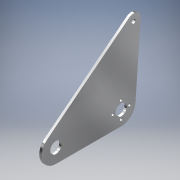
# Autodesk Inventor part: Module Plate
Saved by Autodesk Inventor 2019.4 (Build 234330000, 330)
## iProperties
Created: 2019-12-31
Part Number: Module Plate
Material: Aluminum 6061
Document SubType Name: Modeling
Designer: Mark
Mass: 136.058 g
Surface Area: 235.603 cm^2
Volume: 50.392 cm^3
Density: 2.7 g/cm^3
Appearance: Aluminum - Flat
Author: Mark
Autodesk Inventor part; units mm, degrees
ref_plane "YZ Plane" through (0, 0, 0) normal (1, 0, 0) x (0, 1, 0)
ref_plane "XZ Plane" through (0, 0, 0) normal (0, 1, 0) x (-1, 0, 0)
ref_plane "XY Plane" through (0, 0, 0) normal (0, 0, 1) x (1, 0, 0)
sketch "Sketch1" plane through (0, 0, 0) normal (1, 0, 0) x (0, 1, 0)
  circle A0 centre (0, 0) radius 12
  circle A1 centre (0, -137.4) radius 12
  line L0 (0, 0) -> (0, -137.4)
  line L1 (0, 0) -> (137.4, 0) construction
  line L2 (0, 0) -> (0, -137.4) construction
  line L3 (-30, 0) -> (-30, -137.4)
  line L4 (30, -137.4) -> (30, 0)
  arc A2 (30, 0) -> (-30, 0) centre (0, 0) ccw
  arc A3 (-30, -137.4) -> (30, -137.4) centre (0, -137.4) ccw
  circle A4 centre (0, -137.4) radius 17.5 construction
  line L5 (0, -137.4) -> (17.5, -137.4) construction
  line L6 (0, -137.4) -> (17.5, -137.4) construction
  circle A5 centre (17.5, -137.4) radius 2.65
  line L7 (0, -137.4) -> (0, -119.9) construction
  circle A6 centre (0, -119.9) radius 2.65
  line L8 (0, -137.4) -> (-17.5, -137.4) construction
  circle A7 centre (-17.5, -137.4) radius 2.65
  line L9 (0, -137.4) -> (0, -154.9) construction
  circle A8 centre (0, -154.9) radius 2.65
  line L10 (0, -137.4) -> (147.7212, -163.4472) construction
  line L11 (0, -137.4) -> (150, -137.4) construction
  circle A9 centre (147.7212, -163.4472) radius 5.1
  arc A10 (146.6067, -178.4058) -> (159.5086, -154.1705) centre (147.7212, -163.4472) ccw
  line L12 (146.6067, -178.4058) -> (-2.2289, -167.3171)
  line L13 (159.5086, -154.1705) -> (23.5748, 18.5534)
  point P0 (0, -68.7)
  point P1 (-20.8357, -21.5841)
  dimension "d9" = 35
  dimension "d0" = 24
  dimension "d1" = 24
  dimension "d4" = 90
  dimension "d5" = 137.4
  dimension "d6" = 60
  dimension "d10" = 0
  dimension "d11" = 5.3
  dimension "d14" = 360
  dimension "d16" = 150
  dimension "d17" = 350
  dimension "d18" = 10.2
  dimension "d19" = 30
  constraints: 30 end point, 10 centre point, 9 point on circle, 8 tangent, 5 coincident, 3 equal length, 3 horizontal, 2 vertical, 1 horizontal alignment, 1 midpoint, 1 parallel, 23 other
  measures "d0" diameter of A0
  measures "d1" diameter of A1
  measures "d4" angle of L0 L1
  measures "d5" distance of L0.start L0.end
  measures "d6" diameter of A3
  measures "d10" distance between parallel lines of L5 L6
  measures "d11" diameter of A5
  measures "d16" distance of L9.start L10.end
  measures "d18" diameter of A9
  measures "d19" diameter of A10
extrude "Extrusion1" add sketch "Sketch1" along normal blind 5 contours A2 L4 A3 L3 | L13 A10 L12 A3 L4 A2 | A9
sketch "Sketch2" plane through (5, 0, 0) normal (1, 0, 0) x (0, 0, -1)
  circle A0 centre (163.4472, 147.7212) radius 4.25
  arc A1 (178.4058, 146.6067) -> (154.1705, 159.5086) centre (163.4472, 147.7212) ccw projected
  point P0 (0, 0)
  point P1 (17.6579, 112.2275)
  dimension "d20" = 8.5
  constraints: 1 centre point, 2 other
  measures "d20" diameter of A0
extrude "Extrusion2" cut sketch "Sketch2" against normal blind 10
body "Solid1"
